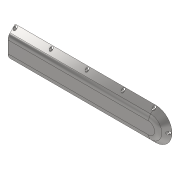
# Autodesk Inventor part: Cover for robot head
Saved by Autodesk Inventor 2020.3 (Build 243373010, 373A)
## iProperties
Created: 2021-04-27
Part Number: Cover for robot head
Material: Steel, Alloy
Document SubType Name: Modeling
Designer: marti
Density: 7.73 g/cm^3
Appearance: Semi-Polished
Author: marti
Autodesk Inventor part; units mm, degrees
ref_plane "YZ Plane" through (0, 0, 0) normal (1, 0, 0) x (0, 1, 0)
ref_plane "XZ Plane" through (0, 0, 0) normal (0, 1, 0) x (-1, 0, 0)
ref_plane "XY Plane" through (0, 0, 0) normal (0, 0, 1) x (1, 0, 0)
sketch "Sketch2" plane through (0, 0, 0) normal (0, 0, 1) x (1, 0, 0)
  circle A0 centre (-43, -20) radius 2.067
  circle A1 centre (-143, -20) radius 2.067
  circle A2 centre (-93, 20) radius 2.067
  circle A3 centre (-193, -20) radius 2.067
  circle A4 centre (20, 0) radius 2.067
  circle A5 centre (0, 20) radius 2.067
  circle A6 centre (-193, 20) radius 2.067
  circle A7 centre (-143, 20) radius 2.067
  circle A8 centre (-43, 20) radius 2.067
  circle A9 centre (-93, -20) radius 2.067
  circle A10 centre (0, -20) radius 2.067
  line L0 (-195.5, -22.5) -> (-195.5, 22.5)
  line L1 (-195.5, -22.5) -> (0, -22.5)
  arc A11 (0, -22.5) -> (0, 22.5) centre (0, 0) ccw
  line L2 (-195.5, 22.5) -> (0, 22.5)
  line L3 (0, -17.5) -> (-190.5, -17.5)
  line L4 (-190.5, -17.5) -> (-190.5, 17.5)
  line L5 (-190.5, 17.5) -> (0, 17.5)
  arc A12 (0, -17.5) -> (0, 17.5) centre (0, 0) ccw
  point P0 (-197.5, 0)
  constraints: 13 centre point, 12 end point, 4 point on circle
extrude "Extrusion1" add sketch "Sketch2" along normal mid plane 10 contours L0 L2 A11 L1 | L3 L4 L5 A12
chamfer "Chamfer1" distance 10 angle 45 3 edges at (-97.75, 22.5, 5) (22.5, 0, 5) (-97.75, -22.5, 5)
fillet "Fillet2" radius 10 3 edges at (-97.75, -12.5, 5) (12.5, 0, 5) (-97.75, 12.5, 5)
body "Solid1"
